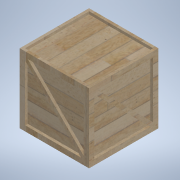
# Autodesk Inventor part: cargoPrototype
Saved by Autodesk Inventor 2020.3 (Build 243373000, 373)
## iProperties
Created: 2021-02-26
Part Number: cargoPrototype
Material: Wood (Maple)
Document SubType Name: Modeling
Designer: con_c_000
Density: 0.67 g/cm^3
Appearance: Natural Maple - Glossy Dark Tint
Author: con_c_000
Autodesk Inventor part; units mm, degrees
ref_plane "YZ Plane" through (0, 0, 0) normal (1, 0, 0) x (0, 1, 0)
ref_plane "XZ Plane" through (0, 0, 0) normal (0, 1, 0) x (-1, 0, 0)
ref_plane "XY Plane" through (0, 0, 0) normal (0, 0, 1) x (1, 0, 0)
sketch "Sketch1" plane through (0, 0, 0) normal (0, 1, 0) x (-1, 0, 0)
  line L0 (158.5647, 157.6724) -> (-146.2353, 157.6724)
  line L1 (-146.2353, 157.6724) -> (-146.2353, -147.1276)
  line L2 (-146.2353, -147.1276) -> (158.5647, -147.1276)
  line L3 (158.5647, -147.1276) -> (158.5647, 157.6724)
  point P0 (0, 0)
  dimension "d0" = 304.8
  dimension "d1" = 304.8
  constraints: 8 end point, 2 parallel, 1 horizontal, 1 perpendicular
  measures "d0" distance of L2.end L1.end
  measures "d1" distance of L1.end L0.end
extrude "Extrusion1" add sketch "Sketch1" along normal blind 304.8
sketch "Sketch2" plane through (146.2353, 0, 157.6724) normal (1, 0, 0) x (0, 0, -1)
  line L0 (-12.7, 317.5) -> (317.5, 317.5)
  line L1 (317.5, 317.5) -> (317.5, -12.7)
  line L2 (317.5, -12.7) -> (-12.7, -12.7)
  line L3 (-12.7, -12.7) -> (-12.7, 317.5)
  line L4 (0, 304.8) -> (304.8, 304.8) projected
  line L5 (0, 0) -> (0, 304.8) projected
  line L6 (12.7, 292.1) -> (292.1, 292.1)
  line L7 (292.1, 292.1) -> (292.1, 12.7)
  line L8 (292.1, 12.7) -> (12.7, 12.7)
  line L9 (12.7, 12.7) -> (12.7, 292.1)
  line L10 (25.4, 292.1) -> (292.1, 25.4)
  line L11 (279.4, 12.7) -> (12.7, 279.4)
  point P0 (157.6724, 0)
  dimension "d4" = 330.2
  dimension "d5" = 330.2
  dimension "d6" = 12.7
  dimension "d7" = 12.7
  dimension "d8" = 25.4
  dimension "d9" = 25.4
  dimension "d10" = 25.4
  dimension "d11" = 25.4
  dimension "d17" = 12.7
  dimension "d18" = 12.7
  dimension "d19" = 12.7
  constraints: 20 end point, 5 parallel, 4 point on line, 2 horizontal, 2 perpendicular
  measures "d4" distance of L1.end L2.end
  measures "d5" distance of L0.end L1.end
  measures "d6" distance between parallel lines of L4 L0
  measures "d7" distance between parallel lines of L5 L3
  measures "d8" distance between parallel lines of L0 L6
  measures "d9" distance between parallel lines of L1 L7
  measures "d10" distance between parallel lines of L9 L3
  measures "d11" distance between parallel lines of L2 L8
  measures "d17" distance of L6.start L10.start
  measures "d18" distance of L7.end L10.end
  measures "d19" distance of L7.end L11.start
extrude "Extrusion2" add sketch "Sketch2" along normal blind 12.7 contours L0 L1 L2 L3 | L6 L10 L7 L8 L11 L9
ref_plane "Work Plane1" through (-6.1647, 0, -147.1276) normal (-1, 0, 0) x (0, 0, 1)
ref_plane "Work Plane2" through (-158.5647, 0, 5.2724) normal (0, 0, 1) x (1, 0, 0)
pattern_circular "Circular Pattern1" count 4 over 360 about axis through (-6.1647, 0, 5.2724) along (0, 1, 0) of "Extrusion2"
body "Solid1"
